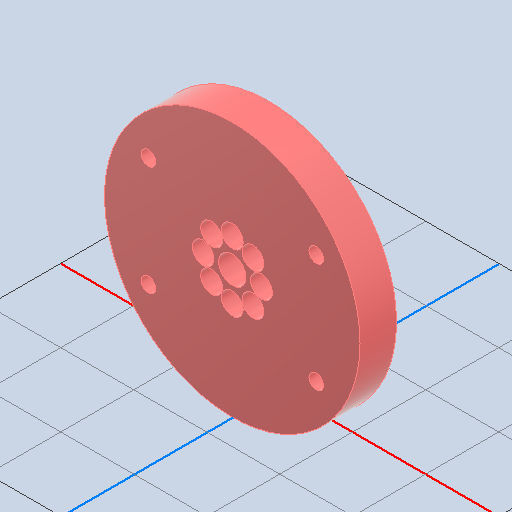
# Autodesk Inventor part: 000.005.004.003 - ПОВОРОТНЫЙ ДИСК
Saved by Autodesk Inventor 2022 (Build 260153000, 153)
## iProperties
Created: 2022-12-17
Part Number: 000.005.004.003 - ПОВОРОТНЫЙ ДИСК
Material: Пластик АБС
Document SubType Name: Modeling
Designer: Petrov Ivan
Density: 1.06 g/cm^3
Appearance: Гладкий — красный
Author: Petrov Ivan
Autodesk Inventor part; units mm, degrees
ref_plane "YZ Plane" through (0, 0, 0) normal (1, 0, 0) x (0, 1, 0)
ref_plane "XZ Plane" through (0, 0, 0) normal (0, 1, 0) x (-1, 0, 0)
ref_plane "XY Plane" through (0, 0, 0) normal (0, 0, 1) x (1, 0, 0)
sketch "Эскиз1" plane through (0, 0, 0) normal (0, 0, 1) x (1, 0, 0)
  circle A0 centre (0, 0) radius 3.75
  circle A1 centre (0, 0) radius 10.8
  circle A2 centre (0, 0) radius 2.85
  circle A3 centre (-5.6569, 5.6569) radius 1.2
  circle A4 centre (-8, 0) radius 1.2
  circle A5 centre (-5.6569, -5.6569) radius 1.2
  circle A6 centre (0, -8) radius 1.2
  circle A7 centre (5.6569, -5.6569) radius 1.2
  circle A8 centre (8, 0) radius 1.2
  circle A9 centre (5.6569, 5.6569) radius 1.2
  circle A10 centre (0, 8) radius 1.2
  circle A11 centre (0, 0) radius 11
  constraints: 12 centre point
extrude "Выдавливание1" add sketch "Эскиз1" along normal blind 3 contours A1 | A11
sketch "Эскиз6" plane through (0, 0, 3) normal (0, 0, 1) x (1, 0, 0)
  circle A0 centre (0, 0) radius 3.75 projected
  circle A1 centre (0, 0) radius 35
  circle A2 centre (0, 0) radius 11 projected
  circle A3 centre (0, 0) radius 3.75 projected
  circle A4 centre (-5.6569, 5.6569) radius 1.2 projected
  circle A5 centre (-8, 0) radius 1.2 projected
  circle A6 centre (-5.6569, -5.6569) radius 1.2 projected
  circle A7 centre (0, -8) radius 1.2 projected
  circle A8 centre (5.6569, -5.6569) radius 1.2 projected
  circle A9 centre (8, 0) radius 1.2 projected
  circle A10 centre (5.6569, 5.6569) radius 1.2 projected
  circle A11 centre (0, 8) radius 1.2 projected
  dimension "d21" = 70
  constraints: 1 centre point, 1 coincident
  measures "d21" diameter of A1
extrude "Выдавливание6" add sketch "Эскиз6" along normal blind 10 contours A1 | A2
sketch "Эскиз7" plane through (0, 0, 13) normal (0, 0, 1) x (1, 0, 0)
  circle A0 centre (0, 8) radius 1.2 projected
  circle A1 centre (0, 8) radius 3
  point P0 (0, 0)
  dimension "d24" = 6
  constraints: 1 centre point, 1 coincident
  measures "d24" diameter of A1
extrude "Выдавливание7" cut sketch "Эскиз7" against normal blind 5 contours A0 | A1
pattern_circular "Круговой массив2" count 8 over 360 about axis through (0, 0, 0) along (0, 0, 1) of "Выдавливание7"
sketch "Эскиз8" plane through (0, 0, 13) normal (0, 0, 1) x (1, 0, 0)
  line L0 (0, 0) -> (-23, 0) construction
  line L1 (-23, 0) -> (-23, 15) construction
  circle A0 centre (-23, 15) radius 2
  dimension "d30" = 23
  dimension "d31" = 15
  dimension "d32" = 4
  constraints: 4 end point, 1 centre point, 1 coincident, 1 horizontal, 1 perpendicular
  measures "d30" distance of L0.start L0.end
  measures "d31" distance of L0.end L1.end
  measures "d32" diameter of A0
extrude "Выдавливание8" cut sketch "Эскиз8" against normal through all
sketch "Эскиз9" plane through (0, 0, 3) normal (0, 0, -1) x (-1, 0, 0)
  circle A0 centre (23, 15) radius 2 projected
  circle A1 centre (23, 15) radius 3
  point P0 (0, 0)
  dimension "d35" = 6
  constraints: 1 centre point, 1 coincident
  measures "d35" diameter of A1
extrude "Выдавливание9" cut sketch "Эскиз9" against normal blind 5 contours A0 | A1
mirror "Зеркальное отражение3" about plane through (0, 0, 0) normal (0, 1, 0) of "Выдавливание9", "Выдавливание8"
mirror "Зеркальное отражение4" about plane through (0, 0, 0) normal (1, 0, 0) of "Выдавливание9", "Зеркальное отражение3", "Выдавливание8"
